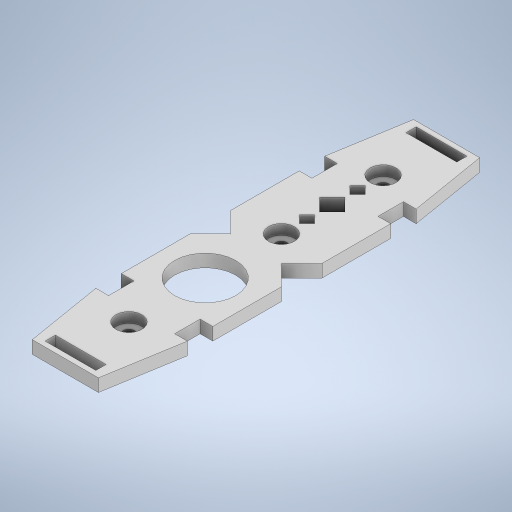
# Autodesk Inventor part: Side w motor
Saved by Autodesk Inventor 2023 (Build 270158000, 158)
## iProperties
Created: 2025-04-09
Part Number: Side w motor
Material: Generic
Document SubType Name: Modeling
Designer: 1khanhan2
Density: 1 g/cm^3
Appearance: Default
Author: 1khanhan2
Autodesk Inventor part; units mm, degrees
ref_plane "YZ Plane" through (0, 0, 0) normal (1, 0, 0) x (0, 1, 0)
ref_plane "XZ Plane" through (0, 0, 0) normal (0, 1, 0) x (-1, 0, 0)
ref_plane "XY Plane" through (0, 0, 0) normal (0, 0, 1) x (1, 0, 0)
sketch "Sketch1" plane through (0, 0, 0) normal (0, 1, 0) x (-1, 0, 0)
  line L0 (36, -30) -> (36, -120)
  line L1 (31, -150) -> (5, -150)
  line L2 (0, -120) -> (0, -30)
  circle A0 centre (18, -25) radius 5.1
  circle A1 centre (18, -55) radius 12
  circle A2 centre (18, -85) radius 5.1
  circle A3 centre (18, -125) radius 5.1
  line L3 (36, -30) -> (31, -30)
  line L4 (31, -30) -> (31, -40)
  line L5 (31, -40) -> (36, -40)
  line L6 (36, -150) -> (36, -120)
  line L7 (36, -120) -> (31, -120)
  line L8 (31, -120) -> (31, -110)
  line L9 (31, -110) -> (36, -110)
  line L10 (0, -30) -> (5, -30)
  line L11 (5, -30) -> (5, -40)
  line L12 (5, -40) -> (0, -40)
  line L13 (0, -120) -> (5, -120)
  line L14 (5, -120) -> (5, -110)
  line L15 (5, -110) -> (0, -110)
  circle A4 centre (18, -25) radius 2.25
  circle A5 centre (18, -85) radius 2.25
  circle A6 centre (18, -125) radius 2.25
  line L16 (31, 0) -> (36, -30)
  line L17 (31, -150) -> (36, -120)
  line L18 (5, 0) -> (0, -30)
  line L19 (5, -150) -> (0, -120)
  line L20 (31, 0) -> (5, 0)
  line L21 (18, -100) -> (23, -105)
  line L22 (18, -110) -> (23, -105)
  line L23 (18, -100) -> (13, -105)
  line L24 (13, -105) -> (18, -110)
  line L25 (21, -95.05) -> (18, -98.05)
  line L26 (18, -98.05) -> (15, -95.05)
  line L27 (18, -92.05) -> (15, -95.05)
  line L28 (18, -92.05) -> (21, -95.05)
  line L29 (21, -114.95) -> (18, -117.95)
  line L30 (18, -117.95) -> (15, -114.95)
  line L31 (15, -114.95) -> (18, -111.95)
  line L32 (18, -111.95) -> (21, -114.95)
  line L33 (31, -150) -> (28, -150)
  line L34 (5, -150) -> (8, -150)
  line L35 (8, -148) -> (28, -148)
  line L36 (28, -148) -> (28, -144)
  line L37 (28, -144) -> (8, -144)
  line L38 (8, -144) -> (8, -148)
  line L39 (31, 0) -> (28, 0)
  line L40 (5, 0) -> (8, 0)
  line L41 (8, -2) -> (28, -2)
  line L42 (28, -2) -> (28, -6.0756)
  line L43 (28, -6.0756) -> (8, -6.0756)
  line L44 (8, -6.0756) -> (8, -2)
  line L45 (36, -75) -> (36, -83)
  line L46 (36, -75) -> (36, -67)
  line L47 (36, -67) -> (28, -75)
  line L48 (36, -83) -> (28, -75)
  line L49 (0, -75) -> (0, -83)
  line L50 (0, -75) -> (0, -67)
  line L51 (0, -67) -> (8, -75)
  line L52 (0, -83) -> (8, -75)
  point P0 (0, 0)
  point P1 (18, 0)
  point P2 (18, -150)
  dimension "d4" = 24
  dimension "d5" = 30
  dimension "d6" = 10.2
  dimension "d7" = 30
  dimension "d8" = 10.2
  dimension "d9" = 40
  dimension "d12" = 5
  dimension "d15" = 5
  dimension "d16" = 10
  dimension "d17" = 5
  dimension "d19" = 4.5
  dimension "d20" = 4.5
  dimension "d25" = 36
  dimension "d36" = 3
  dimension "d37" = 2
  dimension "d39" = 4
  dimension "d41" = 2
  dimension "d42" = 3
  dimension "d45" = 8
  constraints: 106 end point, 16 perpendicular, 16 point on line, 7 centre point, 3 coincident, 3 midpoint, 3 parallel, 1 horizontal, 1 vertical
  measures "d4" diameter of A1
  measures "d5" distance of A1.centre A0.centre
  measures "d6" diameter of A2
  measures "d7" distance of A2.centre A1.centre
  measures "d8" diameter of A3
  measures "d9" distance of A3.centre A2.centre
  measures "d12" distance of L0.start L3.end
  measures "d15" distance of L0.end L7.end
  measures "d16" distance of L7.end L8.end
  measures "d17" distance of L2.end L10.end
  measures "d19" diameter of A5
  measures "d20" diameter of A6
  measures "d25" distance between parallel lines of L2 L0
  measures "d36" distance of L1.start L33.end
  measures "d37" distance of L33.end L35.end
  measures "d39" distance of L35.end L36.end
  measures "d41" distance of L39.end L41.end
  measures "d42" distance of L18.start L40.end
  measures "d45" distance of L49.start L49.end
extrude "Extrusion1" add sketch "Sketch1" along normal blind 5 contours L3 L4 L5 L0 L47 L48 L9 L8 L7 L17 L1 L19 L13 L14 L15 L2 L52 L51 L12 L11 L10 L18 L20 L16
extrude "Extrusion2" add sketch "Sketch1" along normal blind 1 contours A0 | A2 | A3
body "Solid1"
